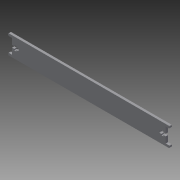
# Autodesk Inventor part: Fin 27270714b
Saved by Autodesk Inventor 2013 (Build 170138000, 138)
## iProperties
Created: 2014-07-01
Part Number: Fin 27270714b
Material: Generic
Document SubType Name: Modeling
Designer: STACKPOLE
Density: 1 g/cm^3
Author: STACKPOLE
Autodesk Inventor part; units mm, degrees
ref_plane "YZ Plane" through (0, 0, 0) normal (1, 0, 0) x (0, 1, 0)
ref_plane "XZ Plane" through (0, 0, 0) normal (0, 1, 0) x (-1, 0, 0)
ref_plane "XY Plane" through (0, 0, 0) normal (0, 0, 1) x (1, 0, 0)
sketch "Sketch1" plane through (0, 0, 0) normal (0, 1, 0) x (-1, 0, 0)
  line L0 (0, 1) -> (0, 2)
  line L1 (1, 3) -> (5, 3)
  line L2 (5, 22) -> (1, 22)
  line L3 (0, 23) -> (0, 24)
  line L4 (1, 25) -> (105, 25)
  line L5 (105, 25) -> (105, 0) construction
  line L6 (105, 0) -> (1, 0)
  line L7 (5, 14) -> (8, 14)
  line L8 (8, 14) -> (8, 15.5)
  line L9 (8, 15.5) -> (10.5, 15.5)
  line L10 (10.5, 9.5) -> (8, 9.5)
  line L11 (8, 9.5) -> (8, 11)
  line L12 (8, 11) -> (5, 11)
  line L13 (5, 3) -> (5, 11)
  line L14 (5, 14) -> (5, 22)
  line L15 (10.5, 14) -> (12.5, 14)
  line L16 (13.5, 13) -> (13.5, 12)
  line L17 (12.5, 11) -> (10.5, 11)
  line L18 (10.5, 15.5) -> (10.5, 14)
  line L19 (10.5, 11) -> (10.5, 9.5)
  arc A0 (1, 25) -> (0, 24) centre (1, 24) ccw
  arc A1 (0, 23) -> (1, 22) centre (1, 23) ccw
  arc A2 (1, 3) -> (0, 2) centre (1, 2) ccw
  arc A3 (0, 1) -> (1, 0) centre (1, 1) ccw
  arc A4 (12.5, 11) -> (13.5, 12) centre (12.5, 12) ccw
  arc A5 (13.5, 13) -> (12.5, 14) centre (12.5, 13) ccw
  line L20 (210, 1) -> (210, 2)
  line L21 (209, 3) -> (205, 3)
  line L22 (205, 22) -> (209, 22)
  line L23 (210, 23) -> (210, 24)
  line L24 (209, 25) -> (105, 25)
  line L25 (105, 0) -> (209, 0)
  line L26 (205, 14) -> (202, 14)
  line L27 (202, 14) -> (202, 15.5)
  line L28 (202, 15.5) -> (199.5, 15.5)
  line L29 (199.5, 9.5) -> (202, 9.5)
  line L30 (202, 9.5) -> (202, 11)
  line L31 (202, 11) -> (205, 11)
  line L32 (196.5, 16) -> (105, 16) construction
  line L33 (205, 3) -> (205, 11)
  line L34 (205, 14) -> (205, 22)
  line L35 (199.5, 14) -> (197.5, 14)
  line L36 (196.5, 13) -> (196.5, 12)
  line L37 (197.5, 11) -> (199.5, 11)
  line L38 (199.5, 15.5) -> (199.5, 14)
  line L39 (199.5, 11) -> (199.5, 9.5)
  arc A6 (210, 24) -> (209, 25) centre (209, 24) ccw
  arc A7 (209, 22) -> (210, 23) centre (209, 23) ccw
  arc A8 (210, 2) -> (209, 3) centre (209, 2) ccw
  arc A9 (209, 0) -> (210, 1) centre (209, 1) ccw
  arc A10 (196.5, 12) -> (197.5, 11) centre (197.5, 12) ccw
  arc A11 (197.5, 14) -> (196.5, 13) centre (197.5, 13) ccw
  point P0 (0, 0)
  point P1 (0, 3)
  point P2 (0, 22)
  point P3 (0, 25)
  point P4 (10.5, 21)
  point P5 (13.5, 14)
  point P6 (13.5, 11)
  point P7 (210, 0)
  point P8 (210, 3)
  point P9 (210, 22)
  point P10 (210, 25)
  point P11 (199.5, 21)
  point P12 (196.5, 14)
  point P13 (196.5, 11)
  dimension "d0" = 3
  dimension "d1" = 5
  dimension "d2" = 19
  dimension "d3" = 3
  dimension "d4" = 105
  dimension "d5" = 5
  dimension "d6" = 6
  dimension "d7" = 2.5
  dimension "d8" = 3
  dimension "d9" = 3
  dimension "d13" = 3
  dimension "d14" = 3
  dimension "d15" = 1
  dimension "d16" = 8.5
  dimension "d17" = 8
  constraints: 80 end point, 37 symmetric about line, 26 point on line, 24 point on circle, 12 centre point, 12 tangent, 11 parallel, 6 perpendicular, 5 equal radius, 3 collinear, 2 horizontal alignment, 2 vertical alignment, 1 vertical, 6 other
  measures "d0" distance of point (0, 0) point (0, 3)
  measures "d1" distance of point (0, 3) L1.end
  measures "d2" distance of L1.end L2.start
  measures "d3" distance of point (0, 22) point (0, 25)
  measures "d4" distance of point (0, 25) L4.end
  measures "d5" distance of L2.start point (0, 22)
  measures "d6" distance of L9.end L10.start
  measures "d7" distance of L8.end L9.end
  measures "d8" distance of L7.start L7.end
  measures "d9" distance between parallel lines of L12 L7
  measures "d13" distance of L15.start point (13.5, 14)
  measures "d14" distance of point (13.5, 11) L17.end
  measures "d15" radius of A0
  measures "d16" distance between parallel lines of L13 L16
  measures "d17" distance of L7.start L2.start
extrude "Extrusion1" add sketch "Sketch1" along normal blind 3
body "Solid1"
